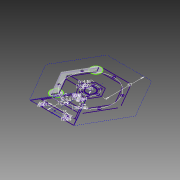
# Autodesk Inventor part: RobotBase
Saved by Autodesk Inventor 2014 SP1 (Build 180222100, 222)
## iProperties
Created: 2015-02-06
Part Number: RobotBase
Material: Glass
Document SubType Name: Modeling
Designer: Erin
Density: 2.18 g/cm^3
Appearance: Clear
Author: Erin
Autodesk Inventor part; units mm, degrees
ref_plane "YZ Plane" through (0, 0, 0) normal (1, 0, 0) x (0, 1, 0)
ref_plane "XZ Plane" through (0, 0, 0) normal (0, 1, 0) x (-1, 0, 0)
ref_plane "XY Plane" through (0, 0, 0) normal (0, 0, 1) x (1, 0, 0)
sketch "Sketch1" plane through (0, 0, 0) normal (0, 0, 1) x (1, 0, 0)
  circle A0 centre (0, 0) radius 7.5
  line L0 (-21.2869, 0) -> (22.3896, 0) construction
  line L1 (0, 21.9302) -> (0, -69.0741) construction
  line L2 (24.9778, -67) -> (-24.9778, -67) construction
  line L3 (-17.5, -57) -> (17.5, -57)
  line L4 (17.5, -57) -> (17.5, -67)
  line L5 (17.5, -67) -> (-17.5, -67)
  line L6 (-17.5, -67) -> (-17.5, -57)
  line L7 (-37.5278, -67) -> (-18.5, -67)
  line L8 (-18.5, -67) -> (-18.5, -56)
  line L9 (-17.5, -62) -> (17.5, -62) construction
  line L10 (-18.5, -59) -> (-22.5, -59)
  line L11 (-22.5, -59) -> (-22.5, -65)
  line L12 (-22.5, -65) -> (-18.5, -65)
  line L13 (-18.5, -65) -> (-18.5, -59)
  line L14 (-17.5, -60) -> (-21.5, -60)
  line L15 (-21.5, -60) -> (-21.5, -64)
  line L16 (-21.5, -64) -> (-17.5, -64)
  line L17 (-17.5, -64) -> (-17.5, -60)
  line L18 (-18.5, -56) -> (-28.8675, -56)
  line L19 (17.5, -60) -> (21.5, -60)
  line L20 (21.5, -60) -> (21.5, -64)
  line L21 (21.5, -64) -> (17.5, -64)
  line L22 (17.5, -64) -> (17.5, -60)
  line L23 (18.5, -67) -> (18.5, -56)
  line L24 (18.5, -67) -> (37.5278, -67)
  line L25 (18.5, -65) -> (22.5, -65)
  line L26 (22.5, -65) -> (22.5, -59)
  line L27 (22.5, -59) -> (18.5, -59)
  line L28 (18.5, -59) -> (18.5, -65)
  line L29 (18.5, -56) -> (28.8675, -56)
  line L30 (-23.7704, -40) -> (28.6931, -40) construction
  line L31 (-17.1762, -35.75) -> (17.1762, -35.75)
  line L32 (-22.0836, -44.25) -> (22.0836, -44.25)
  circle A1 centre (0, -40) radius 2.25
  line L33 (-7.5, -16) -> (7.5, -16)
  line L34 (7.5, -16) -> (7.5, -21)
  line L35 (7.5, -26) -> (-7.5, -26)
  line L36 (-7.5, -26) -> (-7.5, -24)
  line L37 (7.5, -21) -> (-7.5, -21) construction
  line L38 (-7.5, -18) -> (-3.5, -18)
  line L39 (-3.5, -18) -> (-3.5, -21)
  line L40 (-3.5, -24) -> (-7.5, -24)
  line L41 (-7.5, -24) -> (-7.5, -23)
  line L42 (-8.5, -19) -> (-4.5, -19)
  line L43 (-4.5, -19) -> (-4.5, -23)
  line L44 (-4.5, -23) -> (-8.5, -23)
  line L45 (-8.5, -23) -> (-8.5, -19)
  line L46 (7.5, -18) -> (3.5, -18)
  line L47 (3.5, -18) -> (3.5, -21)
  line L48 (3.5, -24) -> (7.5, -24)
  line L49 (7.5, -24) -> (7.5, -18)
  line L50 (8.5, -19) -> (4.5, -19)
  line L51 (4.5, -19) -> (4.5, -23)
  line L52 (4.5, -23) -> (8.5, -23)
  line L53 (8.5, -23) -> (8.5, -19)
  line L54 (-9.815, -19) -> (-31.1769, -56)
  line L55 (-7.5056, -19) -> (-28.8675, -56)
  line L56 (7.5056, -19) -> (28.8675, -56)
  line L57 (-4.5, -21) -> (-8.5, -21)
  line L58 (4.5, -21) -> (8.5, -21)
  line L59 (-21.5, -62) -> (-17.5, -62)
  line L60 (17.5, -62) -> (21.5, -62)
  line L61 (-22.5, -62) -> (-18.5, -62)
  line L62 (22.5, -62) -> (18.5, -62)
  line L63 (-7.5, -21) -> (-3.5, -21)
  line L64 (3.5, -21) -> (7.5, -21)
  line L65 (-28.8675, -56) -> (-31.1769, -56)
  line L66 (28.8675, -56) -> (31.1769, -56)
  line L67 (-10.8853, -24.8539) -> (-12.6173, -23.8539)
  line L68 (10.8875, -24.8576) -> (12.6195, -23.8576)
  line L69 (7.5, -23) -> (7.5, -24)
  line L70 (-7.5, -23) -> (-7.5, -21)
  line L71 (-7.5, -24) -> (-7.5, -16)
  line L72 (7.5, -24) -> (7.5, -26)
  line L73 (-7.5, -21) -> (-7.5, -18)
  line L74 (-3.5, -21) -> (-3.5, -24)
  line L75 (3.5, -21) -> (3.5, -24)
  line L76 (7.5, -21) -> (7.5, -23)
  line L77 (-18.4752, 0) -> (-9.2376, 16)
  line L78 (-9.2376, 16) -> (9.2376, 16)
  line L79 (9.2376, 16) -> (18.4752, 0)
  line L80 (18.4752, 0) -> (9.2376, -16)
  line L81 (9.2376, -16) -> (-9.2376, -16)
  line L82 (-9.2376, -16) -> (-18.4752, 0)
  line L83 (-77.3649, 0) -> (-38.6825, 67) construction
  line L84 (-38.6825, 67) -> (38.6825, 67) construction
  line L85 (38.6825, 67) -> (77.3649, 0) construction
  line L86 (77.3649, 0) -> (38.6825, -67) construction
  line L87 (38.6825, -67) -> (-38.6825, -67) construction
  line L88 (-38.6825, -67) -> (-77.3649, 0) construction
  line L89 (-9.2376, -16) -> (-38.6825, -67) construction
  line L90 (9.2376, -16) -> (38.6825, -67) construction
  line L91 (0, -16.7974) -> (0, -26) construction
  line L92 (9.815, -19) -> (31.1769, -56)
  line L93 (-8.5, -19) -> (-9.815, -19)
  line L94 (8.5, -19) -> (9.815, -19)
  line L95 (-8.5, -23) -> (-9.815, -23)
  line L96 (8.5, -23) -> (9.815, -23)
  line L97 (-31.1769, -56) -> (-37.5278, -67)
  line L98 (31.1769, -56) -> (37.5278, -67)
  circle A2 centre (12.25, 0) radius 2.25
  circle A3 centre (6.125, 10.6088) radius 2.25
  circle A4 centre (-6.125, 10.6088) radius 2.25
  circle A5 centre (-12.25, 0) radius 2.25
  circle A6 centre (-6.125, -10.6088) radius 2.25
  circle A7 centre (6.125, -10.6088) radius 2.25
  line L99 (22.3723, -32.75) -> (39.5485, -3)
  line L100 (27.2798, -41.25) -> (49.3634, -3)
  circle A8 centre (34.641, -20) radius 2.25
  line L101 (39.5485, 3) -> (22.3723, 32.75)
  line L102 (49.3634, 3) -> (27.2798, 41.25)
  circle A9 centre (34.641, 20) radius 2.25
  line L103 (17.1762, 35.75) -> (-17.1762, 35.75)
  line L104 (22.0836, 44.25) -> (-22.0836, 44.25)
  circle A10 centre (0, 40) radius 2.25
  line L105 (-22.3723, 32.75) -> (-39.5485, 3)
  line L106 (-27.2798, 41.25) -> (-49.3634, 3)
  circle A11 centre (-34.641, 20) radius 2.25
  line L107 (-39.5485, -3) -> (-22.3723, -32.75)
  line L108 (-49.3634, -3) -> (-27.2798, -41.25)
  circle A12 centre (-34.641, -20) radius 2.25
  line L109 (22.3723, -32.75) -> (27.2798, -41.25)
  line L110 (49.3634, -3) -> (51.0955, 0)
  line L111 (49.3634, 3) -> (51.0955, 0)
  line L112 (39.5485, -3) -> (41.2805, 0)
  line L113 (39.5485, 3) -> (41.2805, 0)
  line L114 (7.3612, 4.25) -> (38.8268, 4.25)
  line L115 (7.3612, -4.25) -> (38.8268, -4.25)
  arc A13 (8.5, 0) -> (7.3612, 4.25) centre (0, 0) ccw
  arc A14 (7.3612, -4.25) -> (8.5, 0) centre (0, 0) ccw
  arc A15 (7.3612, 4.25) -> (7.3612, -4.25) centre (0, 0) ccw
  line L116 (22.3723, 32.75) -> (27.2798, 41.25)
  circle A16 centre (26.0807, 34.891) radius 8.782
  circle A17 centre (26.0807, -34.1103) radius 9.356
  point P0 (0, -57)
  point P1 (0, -67)
  point P2 (0, -62)
  point P3 (0, -21)
  dimension "d0" = 15
  dimension "d16" = 10
  dimension "d20" = 6
  dimension "d21" = 4
  dimension "d22" = 4
  dimension "d23" = 1
  dimension "d24" = 1
  dimension "d25" = 35
  dimension "d27" = 3
  dimension "d28" = 4
  dimension "d29" = 1
  dimension "d30" = 6
  dimension "d31" = 4
  dimension "d32" = 1
  dimension "d34" = 3
  dimension "d35" = 27
  dimension "d39" = 4.5
  dimension "d41" = 2
  dimension "d42" = 2
  dimension "d44" = 10
  dimension "d45" = 4
  dimension "d46" = 6
  dimension "d48" = 4
  dimension "d49" = 1
  dimension "d50" = 4
  dimension "d52" = 6
  dimension "d53" = 4
  dimension "d54" = 4
  dimension "d55" = 1
  dimension "d56" = 4
  dimension "d57" = 15
  dimension "d60" = 2
  dimension "d81" = 16
  dimension "d83" = 67
  dimension "d84" = 1
  dimension "d86" = 2
  dimension "d87" = 1
  dimension "d88" = 5
  dimension "d89" = 3
  dimension "d90" = 3
  dimension "d112" = 4.5
  dimension "d113" = 2.5
  dimension "d116" = 360
  dimension "d120" = 360
  dimension "d122" = 2
  dimension "d123" = 2
  dimension "d124" = 1
  constraints: 234 end point, 57 parallel, 34 point on line, 26 perpendicular, 18 centre point, 17 midpoint, 12 horizontal, 10 collinear, 8 horizontal alignment, 6 point on circle, 5 coincident, 2 vertical alignment, 1 vertical, 90 other
  measures "d0" diameter of A0
  measures "d16" distance of L5.end L3.start
  measures "d20" distance of L10.end L11.end
  measures "d21" distance of L11.end L12.end
  measures "d22" distance of L14.end L15.end
  measures "d23" distance between parallel lines of L11 L15
  measures "d24" distance between parallel lines of L6 L8
  measures "d25" distance of L3.start L3.end
  measures "d27" distance between parallel lines of L10 L18
  measures "d28" distance of L19.end L20.end
  measures "d29" distance between parallel lines of L4 L23
  measures "d30" distance of L25.end L26.end
  measures "d31" distance of L25.start L25.end
  measures "d32" distance between parallel lines of L20 L26
  measures "d34" distance between parallel lines of L29 L27
  measures "d35" distance between parallel lines of L30 L2
  measures "d39" diameter of A1
  measures "d41" distance edge to line of A1 L31
  measures "d42" distance edge to line of A1 L32
  measures "d44" distance of L33.end L35.start
  measures "d45" distance of L40.start L36.end
  measures "d46" distance of L38.end L40.start
  measures "d48" distance of L42.start L42.end
  measures "d49" distance between parallel lines of L43 L39
  measures "d50" distance of L42.end L43.end
  measures "d52" distance of L46.end L48.start
  measures "d53" distance of L46.start L46.end
  measures "d54" distance of L50.end L51.end
  measures "d55" distance between parallel lines of L47 L51
  measures "d56" distance of L50.start L50.end
  measures "d57" distance of L35.start L35.end
  measures "d60" distance between parallel lines of L54 L55
  measures "d81" distance between parallel lines of L78 L0
  measures "d83" distance between parallel lines of L84 L0
  measures "d84" distance between parallel lines of L89 L54
  measures "d86" distance between parallel lines of L56 L92
  measures "d87" distance between parallel lines of L90 L92
  measures "d88" distance between parallel lines of L37 L33
  measures "d89" distance between parallel lines of L64 L48
  measures "d90" distance between parallel lines of L63 L40
  measures "d112" diameter of A2
  measures "d122" distance edge to line of A2 L115
  measures "d123" distance edge to line of A2 L114
  measures "d124" radial gap between concentric circles of A13 A0
extrude "Extrusion8" add sketch "Sketch1" against normal blind 2 contours A17 L100 L109 L99 | L99 L112 L113 L101 A16 L102 L111 L110 L100 A17 | A16 L101 L116 L102 picked at (27.7457, 34.7764)
extrude "Extrusion9" add sketch "Sketch1" against normal blind 0.3 contours A17 L31 L56 | L56 A17 L92 | L92 A17 L99 L109 L100 | A17 L56 L31 | A17 L100 L109 L99 | A16 L101 L116 L102 | L102 L116 L101 A16
equation "\"d20\" = hinge_w"
equation "\"d21\" = hinge_d"
equation "\"d22\" = hinge_w - 2 * hinge_sp"
equation "\"d23\" = hinge_sp"
equation "\"d24\" = sp"
equation "\"d28\" = hinge_w - 2 * hinge_sp"
equation "\"d29\" = sp"
equation "\"d30\" = hinge_w"
equation "\"d31\" = hinge_d"
equation "\"d32\" = hinge_sp"
equation "\"d39\" = screw"
equation "\"d45\" = hinge_d"
equation "\"d46\" = hinge_w"
equation "\"d48\" = hinge_d"
equation "\"d49\" = hinge_sp"
equation "\"d50\" = hinge_w - 2 * hinge_sp"
equation "\"screw\" = 4.5"
equation "\"k\" = 0.4"
equation "\"sp\" = 1"
equation "\"d14\" = sp"
equation "\"d15\" = sp"
equation "\"d19\" = sp"
equation "\"hinge_d\" = 4"
equation "\"hinge_w\" = 6"
equation "\"hinge_sp\" = 1"
body "Solid11"
